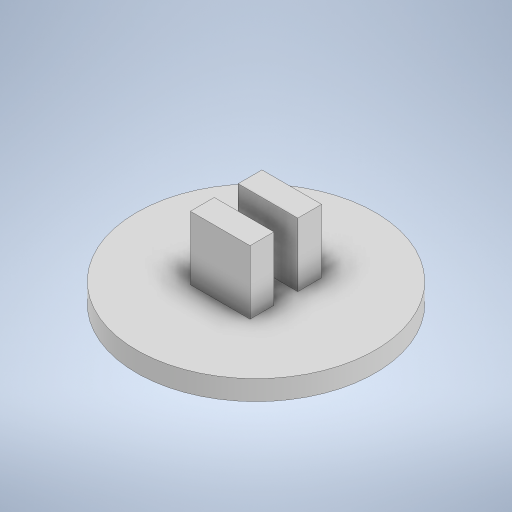
# Autodesk Inventor part: Arm holder
Saved by Autodesk Inventor 2023.2 (Build 272271000, 271)
## iProperties
Created: 2022-12-06
Part Number: Arm holder
Material: Generic
Document SubType Name: Modeling
Designer: Team 4026
Density: 1 g/cm^3
Appearance: Default
Author: Team 4026
Autodesk Inventor part; units mm, degrees
ref_plane "YZ Plane" through (0, 0, 0) normal (1, 0, 0) x (0, 1, 0)
ref_plane "XZ Plane" through (0, 0, 0) normal (0, 1, 0) x (-1, 0, 0)
ref_plane "XY Plane" through (0, 0, 0) normal (0, 0, 1) x (1, 0, 0)
sketch "Sketch1" plane through (0, 0, 0) normal (0, 1, 0) x (-1, 0, 0)
  circle A0 centre (-8.8965, -11.7009) radius 38.1
  point P0 (0, 0)
  dimension "d0" = 76.2
  constraints: 1 centre point
  measures "d0" diameter of A0
extrude "Extrusion1" add sketch "Sketch1" along normal blind 6.35
sketch "Sketch7" plane through (8.8965, 6.35, -11.7009) normal (0, 1, 0) x (1, 0, 0)
  line L0 (9.525, -11.43) -> (-9.525, -11.43) construction
  line L1 (-9.525, -11.43) -> (-9.525, 11.43) construction
  line L2 (-9.525, 11.43) -> (9.525, 11.43) construction
  line L3 (9.525, 11.43) -> (9.525, -11.43) construction
  line L4 (-9.525, 11.43) -> (9.525, -11.43) construction
  line L5 (-9.525, -11.43) -> (9.525, 11.43) construction
  circle A0 centre (0, 0) radius 38.1 construction
  line L6 (-38.1, 0) -> (38.1, 0) construction
  line L7 (0, -38.1) -> (0, 38.1) construction
  line L8 (-9.525, 11.43) -> (9.525, 11.43)
  line L9 (9.525, 11.43) -> (9.525, 3.81)
  line L10 (9.525, 3.81) -> (-9.525, 3.81)
  line L11 (-9.525, 3.81) -> (-9.525, 11.43)
  line L12 (-9.525, -11.43) -> (9.525, -11.43)
  line L13 (9.525, -11.43) -> (9.525, -3.81)
  line L14 (9.525, -3.81) -> (-9.525, -3.81)
  line L15 (-9.525, -3.81) -> (-9.525, -11.43)
  point P0 (-8.8965, -11.7009)
  point P1 (0, 0)
  dimension "d22" = 19.05
  dimension "d23" = 22.86
  dimension "d25" = 7.62
  dimension "d26" = 7.62
  constraints: 32 end point, 6 parallel, 5 perpendicular, 4 midpoint, 4 point on circle, 3 horizontal, 2 point on line, 1 coincident
  measures "d22" distance of L1.end L2.end
  measures "d23" distance of L0.end L1.end
  measures "d25" distance of L8.end L9.end
  measures "d26" distance of L13.end L12.end
extrude "Extrusion3" add sketch "Sketch7" along normal blind 20.32
body "Solid1"
